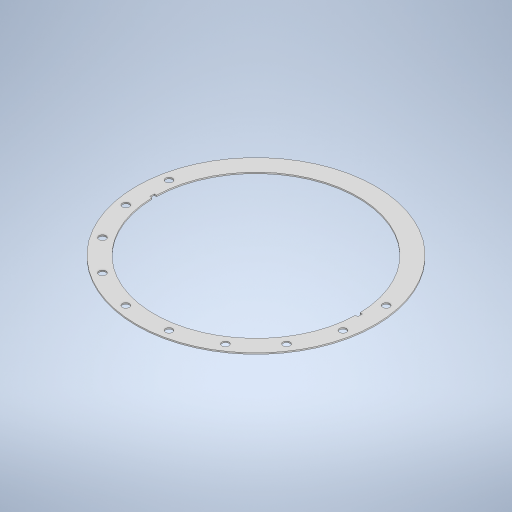
# Autodesk Inventor part: ДМС 011 кольцо под шпильки зад
Saved by Autodesk Inventor 2024.2 (Build 282272000, 272)
## iProperties
Created: 2024-04-23
Part Number: ДМС 011 кольцо под шпильки зад
Material: Generic
Document SubType Name: Sheet Metal
Designer: admin
Density: 1 g/cm^3
Appearance: Default
Sheet Metal Rule: Default
Author: admin
Autodesk Inventor part; units mm, degrees
ref_plane "YZ Plane" through (0, 0, 0) normal (1, 0, 0) x (0, 1, 0)
ref_plane "XZ Plane" through (0, 0, 0) normal (0, 1, 0) x (-1, 0, 0)
ref_plane "XY Plane" through (0, 0, 0) normal (0, 0, 1) x (1, 0, 0)
sketch "Sketch1" plane through (0, 0, 0) normal (0, 0, 1) x (1, 0, 0)
  circle A0 centre (0, 0) radius 230
  circle A1 centre (0, 0) radius 270
  circle A2 centre (0, 0) radius 250 construction
  line L0 (0, 270) -> (0, 230) construction
  point P0 (0, 250)
  dimension "d9" = 500
  dimension "d11" = 40
extrude "Plate1" add sketch "Sketch1" along normal blind 3
sketch "Sketch2" plane through (0, 0, 3) normal (0, 0, 1) x (1, 0, 0)
  circle A0 centre (0, 0) radius 230 construction
  circle A1 centre (0, 0) radius 270 construction
  circle A2 centre (0, 0) radius 270 projected
  circle A3 centre (0, 0) radius 230 projected
  line L0 (0, 0) -> (0, -270) construction
  line L1 (0, 0) -> (-52.6744, -264.812) construction
  line L2 (-44.8708, -225.5806) -> (-52.6744, -264.812) construction
  circle A4 centre (-48.7726, -245.1963) radius 8
  dimension "d20" = 11.25
  dimension "d21" = 16
  constraints: 6 end point, 2 point on circle, 1 centre point, 1 collinear, 1 midpoint, 1 point on line, 1 vertical, 2 other
  measures "d20" angle of L0 L1
  measures "d21" diameter of A4
extrude "Extrusion1" cut sketch "Sketch2" against normal through all contours A4
sketch "Sketch3" plane through (0, 0, 3) normal (0, 0, 1) x (1, 0, 0)
  circle A0 centre (0, 0) radius 230 projected
  line L0 (-230, 0) -> (-235, 0) construction
  line L1 (-235, 5) -> (-235, -5)
  line L2 (-235, 5) -> (-229.9456, 5)
  line L3 (-235, -5) -> (-229.9456, -5)
  line L4 (230, 0) -> (235, 0) construction
  line L5 (235, 5) -> (235, -5)
  line L6 (235, 5) -> (229.9456, 5)
  line L7 (235, -5) -> (229.9456, -5)
  dimension "d23" = 5
  dimension "d24" = 10
  constraints: 16 end point, 6 horizontal, 6 point on circle, 2 equal length, 2 horizontal alignment, 2 midpoint, 2 vertical
  measures "d23" distance of L0.end L0.start
  measures "d24" distance of L1.start L1.end
extrude "Extrusion2" cut sketch "Sketch3" against normal through all contours A0 L6 L5 L7 | A0 L3 L1 L2
pattern_circular "Circular Pattern2" count 10 over 202.5 about axis through (0, 0, 0) along (0, 0, 1) of "Extrusion1" both ways yes
equation "\"d9\" = Шпил_пласт_диам_центров_зад"
equation "\"d11\" = Шпил_пласт_ширина_зад"
equation "\"d21\" = Шпил_пласт_диам_шпильки_зад"
equation "\"d2\" = Thickness"
equation "\"BendRadius\" = Thickness"
equation "\"BendReliefWidth\" = Thickness"
equation "\"BendReliefDepth\" = 0.5 * Thickness"
equation "\"CornerReliefSize\" = 4 * Thickness"
equation "\"MinimumRemnant\" = 2 * Thickness"
equation "\"TransitionRadius\" = BendRadius"
equation "\"JacobiRadiusSize\" = BendRadius"
equation "\"GapSize\" = Thickness"
equation "\"Шпил_пласт_диам_центров_зад\" = 500"
equation "\"Шпил_пласт_ширина_зад\" = 40"
equation "\"Шпил_пласт_диам_шпильки_зад\" = 16"
equation "\"Thickness\" = 3"
body "Solid1"
